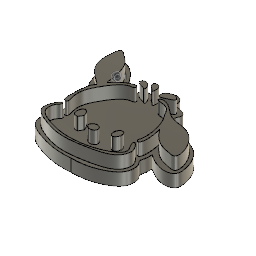
pochacco v3 (Autodesk Fusion 360 design; units mm, degrees)
Autodesk Fusion 360 part; units mm, degrees
(part 1 of 2)
sketch "Sketch1" plane through (0, 0, 0) normal (0, 0, 1) x (1, 0, 0)
  spline S0 degree 5 poles (-0.6709, -13.445) (-0.783, -13.4498) (-1.0072, -13.459) (-1.3442, -13.4715) (-1.7958, -13.4859) (-2.365, -13.4975) (-2.9391, -13.4984) (-3.5187, -13.4833) (-4.106, -13.4469) (-4.7062, -13.3844) (-5.3283, -13.2926) (-5.9822, -13.1694) (-6.6768, -13.0129) (-7.4173, -12.8216) (-8.2027, -12.5932) (-9.0235, -12.3247) (-9.8597, -12.0116) (-10.6769, -11.6473) (-11.4304, -11.2245) (-12.0725, -10.7371) (-12.5591, -10.1826) (-12.8561, -9.5641) (-12.9463, -8.892) (-12.8356, -8.1865) (-12.5616, -7.4801) (-12.1923, -6.8157) (-11.8085, -6.235) (-11.4898, -5.7696) (-11.2987, -5.4297) (-11.2671, -5.1966) (-11.3773, -5.0079) (-11.5611, -4.7626) (-11.7362, -4.3632) (-11.8325, -3.7477) (-11.8251, -2.9297) (-11.7255, -1.9782) (-11.5691, -0.9945) (-11.4045, -0.0892) (-11.2826, 0.6397) (-11.2442, 1.1314) (-11.3109, 1.3806) (-11.4696, 1.4712) (-11.6758, 1.5583) (-11.8871, 1.7597) (-12.0894, 2.0706) (-12.2879, 2.4194) (-12.4965, 2.7197) (-12.728, 2.9335) (-12.9875, 3.0981) (-13.2749, 3.2834) (-13.5856, 3.566) (-13.912, 3.9925) (-14.2441, 4.5797) (-14.5698, 5.3213) (-14.8753, 6.1921) (-15.1462, 7.1536) (-15.3673, 8.1587) (-15.5233, 9.1573) (-15.5998, 10.1003) (-15.5828, 10.9464) (-15.4608, 11.6626) (-15.2255, 12.2237) (-14.8731, 12.6119) (-14.4066, 12.8168) (-13.8357, 12.8345) (-13.1799, 12.6674) (-12.4665, 12.3245) (-11.7278, 11.8208) (-10.9984, 11.1782) (-10.3118, 10.4256) (-9.698, 9.5988) (-9.1805, 8.7406) (-8.7731, 7.9018) (-8.4778, 7.1402) (-8.2807, 6.5221) (-8.1557, 6.1073) (-8.0671, 5.9319) (-7.9735, 5.9948) (-7.8294, 6.2361) (-7.593, 6.5406) (-7.2472, 6.7929) (-6.8148, 6.9181) (-6.383, 6.9377) (-6.0614, 6.9338) (-5.9338, 7.0029) (-6.0018, 7.2066) (-6.1645, 7.543) (-6.2897, 7.972) (-6.2688, 8.4304) (-6.0758, 8.8508) (-5.7419, 9.1752) (-5.3303, 9.3696) (-4.9133, 9.4359) (-4.5448, 9.4322) (-4.2529, 9.4431) (-4.0374, 9.5402) (-3.8635, 9.7382) (-3.6665, 9.976) (-3.3863, 10.167) (-2.9979, 10.2378) (-2.5366, 10.1656) (-2.0673, 9.9643) (-1.6593, 9.6771) (-1.3617, 9.3669) (-1.1717, 9.1088) (-1.0427, 8.9709) (-0.9073, 8.9925) (-0.6976, 9.157) (-0.3587, 9.4027) (0.1403, 9.6505) (0.7963, 9.8245) (1.5579, 9.8797) (2.3378, 9.8023) (3.0366, 9.6007) (3.5622, 9.2992) (3.8526, 8.9306) (3.8934, 8.5294) (3.7467, 8.1242) (3.5327, 7.7352) (3.3803, 7.3754) (3.3923, 7.0507) (3.5931, 6.7603) (3.9282, 6.4983) (4.3136, 6.2565) (4.6678, 6.0275) (4.9601, 5.8076) (5.2168, 5.597) (5.4892, 5.3975) (5.8342, 5.2103) (6.2852, 5.0334) (6.85, 4.8615) (7.5179, 4.6873) (8.2646, 4.5017) (9.0581, 4.2949) (9.8636, 4.057) (10.6488, 3.7787) (11.3903, 3.4522) (12.0729, 3.0716) (12.6879, 2.6335) (13.2319, 2.1373) (13.7056, 1.5858) (14.1121, 0.9858) (14.4558, 0.3482) (14.7408, -0.3111) (14.9701, -0.9713) (15.1451, -1.61) (15.2662, -2.2059) (15.332, -2.7413) (15.3397, -3.2051) (15.2847, -3.5952) (15.1607, -3.9217) (14.9606, -4.1992) (14.6768, -4.4397) (14.3026, -4.644) (13.8328, -4.7975) (13.2671, -4.8789) (12.6118, -4.8662) (11.8835, -4.7446) (11.1103, -4.5126) (10.3365, -4.1907) (9.6195, -3.8228) (9.017, -3.4646) (8.5761, -3.1758) (8.321, -3.0107) (8.2437, -3.0092) (8.2866, -3.1872) (8.3535, -3.5308) (8.3608, -4.0006) (8.2888, -4.5302) (8.1739, -5.0419) (8.076, -5.4679) (8.0543, -5.7687) (8.1385, -5.9551) (8.3064, -6.1019) (8.5111, -6.3) (8.7096, -6.603) (8.8732, -7.0146) (8.9811, -7.5114) (9.0199, -8.0542) (8.9803, -8.6054) (8.8551, -9.142) (8.6396, -9.6517) (8.3323, -10.1301) (7.9349, -10.5777) (7.4531, -10.9973) (6.897, -11.39) (6.2807, -11.7543) (5.6208, -12.0873) (4.9348, -12.3852) (4.24, -12.6443) (3.5517, -12.8619) (2.8818, -13.0371) (2.2375, -13.1714) (1.6203, -13.2697) (1.0271, -13.3388) (0.4523, -13.3865) (0.0014, -13.4134) (-0.3348, -13.4302) (-0.5588, -13.4402) (-0.6709, -13.445) knots 0 0 0 0 0 0 0.00512821 0.01025641 0.01538462 0.02051282 0.02564103 0.03076923 0.03589744 0.04102564 0.04615385 0.05128205 0.05641026 0.06153846 0.06666667 0.07179487 0.07692308 0.08205128 0.08717949 0.09230769 0.0974359 0.1025641 0.10769231 0.11282051 0.11794872 0.12307692 0.12820513 0.13333333 0.13846154 0.14358974 0.14871795 0.15384615 0.15897436 0.16410256 0.16923077 0.17435897 0.17948718 0.18461538 0.18974359 0.19487179 0.2 0.20512821 0.21025641 0.21538462 0.22051282 0.22564103 0.23076923 0.23589744 0.24102564 0.24615385 0.25128205 0.25641026 0.26153846 0.26666667 0.27179487 0.27692308 0.28205128 0.28717949 0.29230769 0.2974359 0.3025641 0.30769231 0.31282051 0.31794872 0.32307692 0.32820513 0.33333333 0.33846154 0.34358974 0.34871795 0.35384615 0.35897436 0.36410256 0.36923077 0.37435897 0.37948718 0.38461538 0.38974359 0.39487179 0.4 0.40512821 0.41025641 0.41538462 0.42051282 0.42564103 0.43076923 0.43589744 0.44102564 0.44615385 0.45128205 0.45641026 0.46153846 0.46666667 0.47179487 0.47692308 0.48205128 0.48717949 0.49230769 0.4974359 0.5025641 0.50769231 0.51282051 0.51794872 0.52307692 0.52820513 0.53333333 0.53846154 0.54358974 0.54871795 0.55384615 0.55897436 0.56410256 0.56923077 0.57435897 0.57948718 0.58461538 0.58974359 0.59487179 0.6 0.60512821 0.61025641 0.61538462 0.62051282 0.62564103 0.63076923 0.63589744 0.64102564 0.64615385 0.65128205 0.65641026 0.66153846 0.66666667 0.67179487 0.67692308 0.68205128 0.68717949 0.69230769 0.6974359 0.7025641 0.70769231 0.71282051 0.71794872 0.72307692 0.72820513 0.73333333 0.73846154 0.74358974 0.74871795 0.75384615 0.75897436 0.76410256 0.76923077 0.77435897 0.77948718 0.78461538 0.78974359 0.79487179 0.8 0.80512821 0.81025641 0.81538462 0.82051282 0.82564103 0.83076923 0.83589744 0.84102564 0.84615385 0.85128205 0.85641026 0.86153846 0.86666667 0.87179487 0.87692308 0.88205128 0.88717949 0.89230769 0.8974359 0.9025641 0.90769231 0.91282051 0.91794872 0.92307692 0.92820513 0.93333333 0.93846154 0.94358974 0.94871795 0.95384615 0.95897436 0.96410256 0.96923077 0.97435897 0.97948718 0.98461538 0.98974359 0.99487179 1 1 1 1 1 1
  point P0 (-4.0523, -13.445)
  point P1 (-9.3122, -12.2106)
  point P2 (-12.8546, -8.4535)
  point P3 (-11.2981, -5.2868)
  point P4 (-11.7275, -4.267)
  point P5 (-11.2981, 1.2613)
  point P6 (-11.6738, 1.5833)
  point P7 (-12.4253, 2.6031)
  point P8 (-13.3377, 3.3545)
  point P9 (-15.5383, 9.4732)
  point P10 (-14.1428, 12.801)
  point P11 (-8.7755, 7.8631)
  point P12 (-8, 6)
  point P13 (-7.1653, 6.7896)
  point P14 (-6, 7)
  point P15 (-6.2529, 7.9704)
  point P16 (-5.2331, 9.3659)
  point P17 (-4.106, 9.5269)
  point P18 (-3.4082, 10.1173)
  point P19 (-1.5833, 9.5806)
  point P20 (-1, 9)
  point P21 (0.3489, 9.6879)
  point P22 (3.8376, 8.7755)
  point P23 (3.4082, 7.219)
  point P24 (4.4817, 6.1455)
  point P25 (5.6088, 5.3404)
  point P26 (10, 4)
  point P27 (14.3575, 0.5099)
  point P28 (15.3236, -3.1935)
  point P29 (14.7332, -4.3743)
  point P30 (11.4055, -4.589)
  point P31 (8.2924, -3.0325)
  point P32 (8.3461, -3.6766)
  point P33 (8.0778, -5.7162)
  point P34 (8.3998, -6.1992)
  point P35 (9, -8)
  point P36 (7.6484, -10.8151)
  point P37 (3, -13)
sketch "Sketch2" plane through (0, 0, 0) normal (0, 0, 1) x (1, 0, 0)
  line L0 (-5, -6) -> (-5.5551, -6.9506)
  spline S0 degree 5 poles (-5, -6) (-4.9873, -6.0708) (-4.971, -6.2073) (-4.9739, -6.3935) (-5.0334, -6.5992) (-5.1932, -6.7885) (-5.4235, -6.9202) (-5.703, -7.002) (-6.0043, -7.0264) (-6.297, -6.972) (-6.5506, -6.8162) (-6.7385, -6.5461) (-6.8412, -6.1684) (-6.8505, -5.7228) (-6.7682, -5.2711) (-6.6041, -4.8826) (-6.3745, -4.621) (-6.1008, -4.5319) (-5.8082, -4.6262) (-5.5241, -4.8758) (-5.2754, -5.2304) (-5.1244, -5.5494) (-5.0469, -5.7823) (-5.0127, -5.9292) (-5, -6) knots 0 0 0 0 0 0 0.05 0.1 0.15 0.2 0.25 0.3 0.35 0.4 0.45 0.5 0.55 0.6 0.65 0.7 0.75 0.8 0.85 0.9 0.95 1 1 1 1 1 1
  point P0 (-6.7359, -6.4753)
  point P1 (-6.1992, -4.589)
sketch "Sketch3" plane through (0, 0, 0) normal (0, 0, 1) x (1, 0, 0)
  spline S0 degree 5 poles (2.1201, -6.3602) (2.1016, -6.3367) (2.0689, -6.2938) (2.0317, -6.2416) (2.003, -6.1859) (1.9929, -6.0963) (2.0011, -5.9456) (2.0273, -5.7181) (2.079, -5.4308) (2.1668, -5.1203) (2.3002, -4.8333) (2.4835, -4.6168) (2.7117, -4.5083) (2.9662, -4.5253) (3.2203, -4.6685) (3.4438, -4.9245) (3.6088, -5.2681) (3.6945, -5.665) (3.6932, -6.0738) (3.6098, -6.4503) (3.4578, -6.754) (3.2564, -6.9526) (3.0276, -7.0286) (2.7933, -6.9844) (2.572, -6.8496) (2.3783, -6.6692) (2.2537, -6.5259) (2.1795, -6.4352) (2.1385, -6.3838) (2.1201, -6.3602) knots 0 0 0 0 0 0 0.04 0.08 0.12 0.16 0.2 0.24 0.28 0.32 0.36 0.4 0.44 0.48 0.52 0.56 0.6 0.64 0.68 0.72 0.76 0.8 0.84 0.88 0.92 0.96 1 1 1 1 1 1
  spline S1 degree 5 poles (-1.3687, -8.0778) (-1.4057, -8.0896) (-1.4798, -8.1125) (-1.5911, -8.1441) (-1.7386, -8.1767) (-1.9212, -8.1873) (-2.1006, -8.1533) (-2.2732, -8.0641) (-2.4307, -7.917) (-2.5593, -7.7201) (-2.6431, -7.4883) (-2.6676, -7.2406) (-2.6223, -6.9973) (-2.5042, -6.777) (-2.3206, -6.5934) (-2.0868, -6.456) (-1.8224, -6.3704) (-1.5487, -6.3386) (-1.2858, -6.3594) (-1.0491, -6.4285) (-0.8479, -6.5391) (-0.687, -6.6827) (-0.5678, -6.8493) (-0.49, -7.0283) (-0.4527, -7.2092) (-0.4557, -7.3821) (-0.4983, -7.5387) (-0.5789, -7.6734) (-0.6943, -7.7842) (-0.8387, -7.8742) (-1.0044, -7.9495) (-1.1476, -8.0032) (-1.2577, -8.0415) (-1.3316, -8.0659) (-1.3687, -8.0778) knots 0 0 0 0 0 0 0.033333 0.066667 0.1 0.133333 0.166667 0.2 0.233333 0.266667 0.3 0.333333 0.366667 0.4 0.433333 0.466667 0.5 0.533333 0.566667 0.6 0.633333 0.666667 0.7 0.733333 0.766667 0.8 0.833333 0.866667 0.9 0.933333 0.966667 1 1 1 1 1 1
  spline S2 degree 5 poles (-10, 2) (-10.0186, 2.0485) (-10.069, 2.1405) (-10.1839, 2.2654) (-10.4088, 2.4137) (-10.7729, 2.59) (-11.1764, 2.7771) (-11.5819, 2.9925) (-11.9682, 3.2495) (-12.3265, 3.5579) (-12.6567, 3.9245) (-12.9634, 4.3535) (-13.2526, 4.8472) (-13.5278, 5.4061) (-13.79, 6.0285) (-14.0377, 6.7091) (-14.2669, 7.4384) (-14.4708, 8.2018) (-14.6403, 8.9783) (-14.7636, 9.7401) (-14.826, 10.451) (-14.8115, 11.0694) (-14.7061, 11.5548) (-14.5002, 11.8734) (-14.1909, 12.0038) (-13.7859, 11.9431) (-13.3038, 11.7103) (-12.771, 11.3384) (-12.2177, 10.8682) (-11.6748, 10.3418) (-11.17, 9.7955) (-10.7246, 9.254) (-10.3499, 8.7227) (-10.0484, 8.1935) (-9.816, 7.6518) (-9.644, 7.0825) (-9.5211, 6.4772) (-9.4351, 5.8403) (-9.3756, 5.1968) (-9.3339, 4.5929) (-9.3001, 4.0833) (-9.2609, 3.7215) (-9.1974, 3.5491) (-9.0816, 3.585) (-8.8769, 3.8179) (-8.5525, 4.2132) (-8.0941, 4.7177) (-7.5191, 5.2648) (-6.8724, 5.7825) (-6.2138, 6.2037) (-5.6084, 6.475) (-5.1161, 6.5669) (-4.7812, 6.4823) (-4.6214, 6.2685) (-4.62, 6.0193) (-4.7442, 5.8262) (-4.9631, 5.7204) (-5.2561, 5.6645) (-5.608, 5.5945) (-6.0083, 5.4519) (-6.4492, 5.2073) (-6.9239, 4.8502) (-7.4251, 4.386) (-7.944, 3.8304) (-8.4681, 3.2048) (-8.9805, 2.5312) (-9.4575, 1.8275) (-9.8727, 1.1074) (-10.2004, 0.382) (-10.42, -0.3397) (-10.5193, -1.05) (-10.4991, -1.7411) (-10.376, -2.4049) (-10.1877, -3.0316) (-9.9939, -3.6092) (-9.8584, -4.1238) (-9.8338, -4.5594) (-9.9446, -4.8985) (-10.1731, -5.1223) (-10.4379, -5.2096) (-10.6397, -5.15) (-10.7214, -4.9593) (-10.7167, -4.6912) (-10.6977, -4.4052) (-10.7214, -4.1315) (-10.7948, -3.8513) (-10.8982, -3.5264) (-10.9976, -3.1177) (-11.063, -2.6127) (-11.0729, -2.0241) (-11.0143, -1.3806) (-10.8849, -0.7203) (-10.6939, -0.083) (-10.4631, 0.4963) (-10.2298, 0.9968) (-10.0408, 1.4121) (-9.9613, 1.6796) (-9.9574, 1.8495) (-9.9814, 1.9515) (-10, 2) knots 0 0 0 0 0 0 0.01052632 0.02105263 0.03157895 0.04210526 0.05263158 0.06315789 0.07368421 0.08421053 0.09473684 0.10526316 0.11578947 0.12631579 0.13684211 0.14736842 0.15789474 0.16842105 0.17894737 0.18947368 0.2 0.21052632 0.22105263 0.23157895 0.24210526 0.25263158 0.26315789 0.27368421 0.28421053 0.29473684 0.30526316 0.31578947 0.32631579 0.33684211 0.34736842 0.35789474 0.36842105 0.37894737 0.38947368 0.4 0.41052632 0.42105263 0.43157895 0.44210526 0.45263158 0.46315789 0.47368421 0.48421053 0.49473684 0.50526316 0.51578947 0.52631579 0.53684211 0.54736842 0.55789474 0.56842105 0.57894737 0.58947368 0.6 0.61052632 0.62105263 0.63157895 0.64210526 0.65263158 0.66315789 0.67368421 0.68421053 0.69473684 0.70526316 0.71578947 0.72631579 0.73684211 0.74736842 0.75789474 0.76842105 0.77894737 0.78947368 0.8 0.81052632 0.82105263 0.83157895 0.84210526 0.85263158 0.86315789 0.87368421 0.88421053 0.89473684 0.90526316 0.91578947 0.92631579 0.93684211 0.94736842 0.95789474 0.96842105 0.97894737 0.98947368 1 1 1 1 1 1
  spline S3 degree 5 poles (1, 6) (0.9263, 6.0109) (0.7895, 6.0343) (0.6205, 6.0771) (0.4842, 6.1578) (0.4887, 6.306) (0.668, 6.4812) (0.9946, 6.6344) (1.4281, 6.7112) (1.9261, 6.6683) (2.4575, 6.4946) (3.0012, 6.2043) (3.5444, 5.829) (4.0813, 5.41) (4.6112, 4.9909) (5.1372, 4.6101) (5.6643, 4.2919) (6.1984, 4.0456) (6.7457, 3.8685) (7.3116, 3.7479) (7.9003, 3.6638) (8.5133, 3.5904) (9.1491, 3.4994) (9.8027, 3.3614) (10.4661, 3.1491) (11.1286, 2.8397) (11.7772, 2.4174) (12.3971, 1.8764) (12.9722, 1.2226) (13.485, 0.4774) (13.9176, -0.321) (14.2533, -1.1246) (14.4786, -1.8814) (14.5849, -2.5424) (14.5707, -3.0681) (14.4432, -3.4348) (14.2199, -3.6411) (13.9316, -3.7154) (13.6114, -3.7012) (13.2853, -3.6437) (12.9596, -3.573) (12.6234, -3.5017) (12.2587, -3.4296) (11.8475, -3.346) (11.3819, -3.2332) (10.8645, -3.0705) (10.3054, -2.8387) (9.7219, -2.525) (9.136, -2.1272) (8.5732, -1.6582) (8.061, -1.1516) (7.626, -0.6569) (7.2904, -0.231) (7.0689, 0.0691) (6.9653, 0.194) (6.9691, 0.1095) (7.0534, -0.1966) (7.1826, -0.7135) (7.318, -1.4065) (7.4251, -2.2144) (7.4779, -3.0523) (7.4606, -3.8283) (7.368, -4.4571) (7.2077, -4.8751) (7.0005, -5.0541) (6.783, -5.0174) (6.6072, -4.851) (6.5178, -4.6493) (6.5225, -4.4413) (6.5897, -4.1849) (6.6736, -3.8184) (6.7343, -3.3035) (6.747, -2.642) (6.6972, -1.8607) (6.5805, -1.0045) (6.4002, -0.1272) (6.1658, 0.717) (5.891, 1.4828) (5.5925, 2.1418) (5.2881, 2.6922) (4.9938, 3.1506) (4.7223, 3.5442) (4.4794, 3.9025) (4.2626, 4.2496) (4.0577, 4.5955) (3.8386, 4.9308) (3.5766, 5.2374) (3.2488, 5.4951) (2.8457, 5.6895) (2.3805, 5.8212) (1.8841, 5.9021) (1.4961, 5.9422) (1.2317, 5.9692) (1.0737, 5.9891) (1, 6) knots 0 0 0 0 0 0 0.01111111 0.02222222 0.03333333 0.04444444 0.05555556 0.06666667 0.07777778 0.08888889 0.1 0.11111111 0.12222222 0.13333333 0.14444444 0.15555556 0.16666667 0.17777778 0.18888889 0.2 0.21111111 0.22222222 0.23333333 0.24444444 0.25555556 0.26666667 0.27777778 0.28888889 0.3 0.31111111 0.32222222 0.33333333 0.34444444 0.35555556 0.36666667 0.37777778 0.38888889 0.4 0.41111111 0.42222222 0.43333333 0.44444444 0.45555556 0.46666667 0.47777778 0.48888889 0.5 0.51111111 0.52222222 0.53333333 0.54444444 0.55555556 0.56666667 0.57777778 0.58888889 0.6 0.61111111 0.62222222 0.63333333 0.64444444 0.65555556 0.66666667 0.67777778 0.68888889 0.7 0.71111111 0.72222222 0.73333333 0.74444444 0.75555556 0.76666667 0.77777778 0.78888889 0.8 0.81111111 0.82222222 0.83333333 0.84444444 0.85555556 0.86666667 0.87777778 0.88888889 0.9 0.91111111 0.92222222 0.93333333 0.94444444 0.95555556 0.96666667 0.97777778 0.98888889 1 1 1 1 1 1
  point P0 (2, -6)
  point P1 (2.4958, -4.6427)
  point P2 (3.6229, -5.3941)
  point P3 (3, -7)
  point P4 (-2.2274, -8.0778)
  point P5 (-2.6031, -7)
  point P6 (-1.3687, -6.3602)
  point P7 (-0.5099, -7)
  point P8 (-0.6172, -7.702)
  point P9 (-11.1371, 2.7641)
  point P10 (-12.962, 4.3743)
  point P11 (-14.6795, 9.2586)
  point P12 (-14.2501, 11.9422)
  point P13 (-11.1371, 9.7416)
  point P14 (-9.4732, 6.0919)
  point P15 (-9.2049, 3.6229)
  point P16 (-8.3998, 4.3743)
  point P17 (-4.8574, 6.4676)
  point P18 (-4.6964, 5.9308)
  point P19 (-5.5015, 5.6088)
  point P20 (-8.5071, 3.1399)
  point P21 (-10.3857, -2.2811)
  point P22 (-10, -4.9111)
  point P23 (-10.6004, -5.1258)
  point P24 (-10.7077, -4.4817)
  point P25 (-10.9224, -3.4082)
  point P26 (-10.6004, 0.1342)
  point P27 (0.5099, 6.2529)
  point P28 (1.476, 6.6823)
  point P29 (4.8037, 4.8574)
  point P30 (8.2388, 3.6229)
  point P31 (12.9083, 1.2613)
  point P32 (14.4111, -3.4082)
  point P33 (13.4987, -3.6766)
  point P34 (12.1569, -3.4082)
  point P35 (9, -2)
  point P36 (7.0043, 0.1342)
  point P37 (7.2727, -1.2076)
  point P38 (7, -5)
  point P39 (6.5749, -4.75)
  point P40 (6.6286, -3.9986)
  point P41 (5.8772, 1.476)
  point P42 (4.3207, 4.1596)
  point P43 (3.1935, 5.5015)
sketch "Sketch4" plane through (0, 0, 0) normal (0, 0, 1) x (1, 0, 0)
sketch "Sketch5" plane through (0, 0, 0) normal (0, 0, 1) x (1, 0, 0)
  spline S0 degree 5 poles (-3.5692, 6.8433) (-3.6043, 6.856) (-3.6794, 6.8823) (-3.8061, 6.9223) (-4.0002, 6.9732) (-4.272, 7.0356) (-4.5557, 7.1066) (-4.8314, 7.1988) (-5.078, 7.3226) (-5.2745, 7.4814) (-5.4018, 7.6695) (-5.4448, 7.8747) (-5.3954, 8.08) (-5.2543, 8.2649) (-5.0345, 8.4072) (-4.7587, 8.4857) (-4.4547, 8.4836) (-4.1514, 8.3912) (-3.8746, 8.2093) (-3.6428, 7.9535) (-3.4638, 7.6549) (-3.3387, 7.3522) (-3.2642, 7.085) (-3.2356, 6.8859) (-3.2489, 6.7742) (-3.3043, 6.7465) (-3.3855, 6.7726) (-3.4687, 6.8057) (-3.5341, 6.8305) (-3.5692, 6.8433) knots 0 0 0 0 0 0 0.04 0.08 0.12 0.16 0.2 0.24 0.28 0.32 0.36 0.4 0.44 0.48 0.52 0.56 0.6 0.64 0.68 0.72 0.76 0.8 0.84 0.88 0.92 0.96 1 1 1 1 1 1
  spline S1 degree 5 poles (-2.3348, 7.5947) (-2.3755, 7.6122) (-2.4586, 7.6494) (-2.5874, 7.7111) (-2.7608, 7.8038) (-2.9617, 7.9396) (-3.128, 8.1) (-3.2436, 8.2888) (-3.2975, 8.5047) (-3.2869, 8.7372) (-3.2163, 8.9686) (-3.0952, 9.1773) (-2.9362, 9.3413) (-2.7532, 9.4415) (-2.5592, 9.4651) (-2.3659, 9.4068) (-2.1834, 9.2683) (-2.0206, 9.0585) (-1.8846, 8.7938) (-1.7808, 8.498) (-1.7131, 8.1995) (-1.6841, 7.927) (-1.6952, 7.7058) (-1.7467, 7.5539) (-1.8384, 7.4776) (-1.9688, 7.4687) (-2.1017, 7.5032) (-2.2144, 7.5446) (-2.2941, 7.5772) (-2.3348, 7.5947) knots 0 0 0 0 0 0 0.04 0.08 0.12 0.16 0.2 0.24 0.28 0.32 0.36 0.4 0.44 0.48 0.52 0.56 0.6 0.64 0.68 0.72 0.76 0.8 0.84 0.88 0.92 0.96 1 1 1 1 1 1
  spline S2 degree 5 poles (-0.2415, 7.2727) (-0.2716, 7.2959) (-0.3244, 7.3456) (-0.3814, 7.43) (-0.4115, 7.5603) (-0.373, 7.7488) (-0.2632, 7.9577) (-0.0918, 8.1792) (0.1256, 8.402) (0.3705, 8.613) (0.6245, 8.7989) (0.8722, 8.9479) (1.1039, 9.0515) (1.3196, 9.1067) (1.5282, 9.1159) (1.7407, 9.0844) (1.9647, 9.0188) (2.199, 8.9248) (2.4265, 8.805) (2.6201, 8.6599) (2.7501, 8.4903) (2.7903, 8.2982) (2.7263, 8.0891) (2.5597, 7.8731) (2.3032, 7.6623) (1.9778, 7.4699) (1.6089, 7.3081) (1.2229, 7.1869) (0.8434, 7.1119) (0.4905, 7.0845) (0.1808, 7.1032) (-0.022, 7.1524) (-0.1442, 7.2064) (-0.2115, 7.2495) (-0.2415, 7.2727) knots 0 0 0 0 0 0 0.033333 0.066667 0.1 0.133333 0.166667 0.2 0.233333 0.266667 0.3 0.333333 0.366667 0.4 0.433333 0.466667 0.5 0.533333 0.566667 0.6 0.633333 0.666667 0.7 0.733333 0.766667 0.8 0.833333 0.866667 0.9 0.933333 0.966667 1 1 1 1 1 1
  spline S3 degree 5 poles (-12.0495, 5.7162) (-12.0629, 5.7109) (-12.0919, 5.7054) (-12.1416, 5.7122) (-12.217, 5.7515) (-12.3166, 5.8483) (-12.4109, 5.9864) (-12.4901, 6.1555) (-12.5463, 6.3409) (-12.5746, 6.5236) (-12.5732, 6.6829) (-12.5427, 6.7996) (-12.486, 6.8588) (-12.4086, 6.8526) (-12.3176, 6.7838) (-12.2219, 6.6625) (-12.1304, 6.5043) (-12.0521, 6.3272) (-11.9944, 6.1493) (-11.9628, 5.9865) (-11.9604, 5.8515) (-11.9825, 5.7742) (-12.0117, 5.7367) (-12.0362, 5.7214) (-12.0495, 5.7162) knots 0 0 0 0 0 0 0.05 0.1 0.15 0.2 0.25 0.3 0.35 0.4 0.45 0.5 0.55 0.6 0.65 0.7 0.75 0.8 0.85 0.9 0.95 1 1 1 1 1 1
  spline S4 degree 5 poles (-11.1908, 6.5749) (-11.2139, 6.5864) (-11.261, 6.6157) (-11.3333, 6.6778) (-11.428, 6.7927) (-11.5301, 6.9681) (-11.6027, 7.1489) (-11.6354, 7.3088) (-11.622, 7.4261) (-11.5636, 7.4898) (-11.469, 7.5013) (-11.3514, 7.4697) (-11.2258, 7.4074) (-11.1067, 7.326) (-11.005, 7.2321) (-10.9276, 7.1277) (-10.8787, 7.0133) (-10.8601, 6.8911) (-10.8721, 6.7667) (-10.9138, 6.6532) (-10.9833, 6.5694) (-11.0581, 6.5406) (-11.1223, 6.5466) (-11.1677, 6.5634) (-11.1908, 6.5749) knots 0 0 0 0 0 0 0.05 0.1 0.15 0.2 0.25 0.3 0.35 0.4 0.45 0.5 0.55 0.6 0.65 0.7 0.75 0.8 0.85 0.9 0.95 1 1 1 1 1 1
  spline S5 degree 5 poles (-11.9422, 8.3998) (-11.9584, 8.3921) (-11.9936, 8.3798) (-12.0541, 8.3713) (-12.1463, 8.3815) (-12.27, 8.436) (-12.3903, 8.5354) (-12.4959, 8.678) (-12.5771, 8.8539) (-12.6261, 9.0426) (-12.6383, 9.2187) (-12.6115, 9.3563) (-12.5474, 9.4342) (-12.451, 9.4402) (-12.332, 9.3774) (-12.2028, 9.2594) (-12.0771, 9.1063) (-11.9682, 8.9403) (-11.8873, 8.7815) (-11.842, 8.6427) (-11.8356, 8.5303) (-11.8613, 8.4632) (-11.8964, 8.4261) (-11.926, 8.4075) (-11.9422, 8.3998) knots 0 0 0 0 0 0 0.05 0.1 0.15 0.2 0.25 0.3 0.35 0.4 0.45 0.5 0.55 0.6 0.65 0.7 0.75 0.8 0.85 0.9 0.95 1 1 1 1 1 1
  spline S6 degree 5 poles (-13.284, 9.7416) (-13.303, 9.7417) (-13.3412, 9.7442) (-13.3988, 9.7546) (-13.4718, 9.7822) (-13.5469, 9.8393) (-13.5967, 9.9177) (-13.6147, 10.0137) (-13.5983, 10.1199) (-13.5501, 10.2245) (-13.4765, 10.3138) (-13.3862, 10.3745) (-13.2894, 10.3965) (-13.1956, 10.3753) (-13.1132, 10.3149) (-13.049, 10.2254) (-13.0078, 10.12) (-12.993, 10.0128) (-13.0057, 9.916) (-13.045, 9.8372) (-13.1079, 9.7804) (-13.1731, 9.7534) (-13.2275, 9.7436) (-13.2651, 9.7415) (-13.284, 9.7416) knots 0 0 0 0 0 0 0.05 0.1 0.15 0.2 0.25 0.3 0.35 0.4 0.45 0.5 0.55 0.6 0.65 0.7 0.75 0.8 0.85 0.9 0.95 1 1 1 1 1 1
  spline S7 degree 5 poles (7.6484, 1.3687) (7.6156, 1.3787) (7.5486, 1.4013) (7.4449, 1.4432) (7.3068, 1.5155) (7.1543, 1.6314) (7.0421, 1.7688) (6.9865, 1.9208) (6.9971, 2.0777) (7.072, 2.2262) (7.1986, 2.3508) (7.3579, 2.4361) (7.5284, 2.4699) (7.6904, 2.4453) (7.8299, 2.3638) (7.9418, 2.2368) (8.0262, 2.0812) (8.0872, 1.9163) (8.1298, 1.7602) (8.1582, 1.6267) (8.1732, 1.5207) (8.1728, 1.4413) (8.1534, 1.384) (8.1106, 1.3442) (8.0402, 1.3199) (7.9397, 1.3126) (7.8352, 1.3229) (7.7451, 1.3413) (7.6811, 1.3587) (7.6484, 1.3687) knots 0 0 0 0 0 0 0.04 0.08 0.12 0.16 0.2 0.24 0.28 0.32 0.36 0.4 0.44 0.48 0.52 0.56 0.6 0.64 0.68 0.72 0.76 0.8 0.84 0.88 0.92 0.96 1 1 1 1 1 1
  spline S8 degree 5 poles (10.1173, 0.6709) (10.1051, 0.6727) (10.0792, 0.6727) (10.0354, 0.6631) (9.9673, 0.6381) (9.8721, 0.6152) (9.7774, 0.6296) (9.6963, 0.7018) (9.6421, 0.8318) (9.6265, 0.9991) (9.6582, 1.1721) (9.7409, 1.316) (9.8726, 1.4) (10.0428, 1.4063) (10.2321, 1.3356) (10.4169, 1.2009) (10.5732, 1.0242) (10.6803, 0.832) (10.7247, 0.6509) (10.705, 0.5034) (10.6345, 0.4042) (10.535, 0.3601) (10.4303, 0.3699) (10.3398, 0.4244) (10.2713, 0.5057) (10.2197, 0.5895) (10.1831, 0.6403) (10.1526, 0.6621) (10.1296, 0.6691) (10.1173, 0.6709) knots 0 0 0 0 0 0 0.04 0.08 0.12 0.16 0.2 0.24 0.28 0.32 0.36 0.4 0.44 0.48 0.52 0.56 0.6 0.64 0.68 0.72 0.76 0.8 0.84 0.88 0.92 0.96 1 1 1 1 1 1
  spline S9 degree 5 poles (10.3857, -1.2076) (10.3583, -1.196) (10.3083, -1.1721) (10.2489, -1.1346) (10.199, -1.0806) (10.1662, -1.0001) (10.1396, -0.9003) (10.1017, -0.7802) (10.0548, -0.6507) (10.0216, -0.5346) (10.0313, -0.4572) (10.1085, -0.4401) (10.2615, -0.4935) (10.4712, -0.609) (10.7022, -0.7668) (10.9114, -0.9402) (11.0574, -1.1012) (11.1095, -1.226) (11.0571, -1.3003) (10.9193, -1.3245) (10.7318, -1.308) (10.5759, -1.2736) (10.4728, -1.2419) (10.4131, -1.2193) (10.3857, -1.2076) knots 0 0 0 0 0 0 0.05 0.1 0.15 0.2 0.25 0.3 0.35 0.4 0.45 0.5 0.55 0.6 0.65 0.7 0.75 0.8 0.85 0.9 0.95 1 1 1 1 1 1
  spline S10 degree 5 poles (11.4055, -0.4562) (11.3841, -0.4553) (11.343, -0.4544) (11.2864, -0.4562) (11.2221, -0.4632) (11.1585, -0.4721) (11.1084, -0.4715) (11.0689, -0.4531) (11.0404, -0.4128) (11.027, -0.3527) (11.0342, -0.2788) (11.0674, -0.1998) (11.1298, -0.1255) (11.2202, -0.0656) (11.3335, -0.0284) (11.4617, -0.0199) (11.5951, -0.0432) (11.7227, -0.0969) (11.8336, -0.1745) (11.9175, -0.2642) (11.9658, -0.3522) (11.9731, -0.4254) (11.9379, -0.4742) (11.8638, -0.4956) (11.7605, -0.4946) (11.6404, -0.4804) (11.5415, -0.467) (11.471, -0.4599) (11.4268, -0.4571) (11.4055, -0.4562) knots 0 0 0 0 0 0 0.04 0.08 0.12 0.16 0.2 0.24 0.28 0.32 0.36 0.4 0.44 0.48 0.52 0.56 0.6 0.64 0.68 0.72 0.76 0.8 0.84 0.88 0.92 0.96 1 1 1 1 1 1
  spline S11 degree 5 poles (12.6936, -1.798) (12.6701, -1.7856) (12.6229, -1.7591) (12.5532, -1.7148) (12.467, -1.6488) (12.381, -1.5596) (12.3257, -1.4685) (12.3073, -1.3807) (12.3282, -1.3027) (12.3862, -1.2432) (12.4744, -1.2112) (12.5837, -1.2144) (12.703, -1.2566) (12.8209, -1.3361) (12.9263, -1.4432) (13.0096, -1.5639) (13.0629, -1.682) (13.0806, -1.782) (13.0607, -1.8521) (13.0051, -1.8867) (12.9195, -1.8867) (12.8337, -1.8625) (12.7643, -1.8336) (12.7172, -1.8104) (12.6936, -1.798) knots 0 0 0 0 0 0 0.05 0.1 0.15 0.2 0.25 0.3 0.35 0.4 0.45 0.5 0.55 0.6 0.65 0.7 0.75 0.8 0.85 0.9 0.95 1 1 1 1 1 1
  spline S12 degree 5 poles (-10.3857, -5.7698) (-10.3398, -5.7371) (-10.2551, -5.6872) (-10.1508, -5.6596) (-10.0569, -5.7193) (-10.0064, -5.9255) (-10.0252, -6.1836) (-10.1183, -6.4064) (-10.2816, -6.5568) (-10.4939, -6.6865) (-10.7234, -6.8783) (-10.9336, -7.1979) (-11.0889, -7.6457) (-11.1589, -8.1793) (-11.1218, -8.7333) (-10.969, -9.2401) (-10.7084, -9.6494) (-10.3693, -9.9511) (-9.993, -10.1641) (-9.6211, -10.3237) (-9.2858, -10.4689) (-8.9976, -10.6294) (-8.7386, -10.816) (-8.4751, -11.0267) (-8.1668, -11.251) (-7.7782, -11.4751) (-7.2864, -11.6854) (-6.6784, -11.8686) (-5.9504, -12.0123) (-5.1065, -12.1059) (-4.1574, -12.1411) (-3.1196, -12.1121) (-2.0138, -12.0165) (-0.8638, -11.856) (0.3042, -11.6367) (1.4634, -11.3679) (2.5862, -11.0615) (3.6461, -10.7299) (4.6178, -10.386) (5.4787, -10.041) (6.2093, -9.7039) (6.7943, -9.3803) (7.2236, -9.0707) (7.4929, -8.7704) (7.605, -8.4666) (7.571, -8.1435) (7.4135, -7.7872) (7.1682, -7.3922) (6.8868, -6.9665) (6.6278, -6.5302) (6.4454, -6.1132) (6.3805, -5.7536) (6.4498, -5.4952) (6.6361, -5.3856) (6.9011, -5.4575) (7.2025, -5.7034) (7.5022, -6.073) (7.7678, -6.4984) (7.9755, -6.9141) (8.112, -7.2761) (8.1777, -7.5874) (8.1833, -7.8838) (8.143, -8.2069) (8.0695, -8.581) (7.9678, -8.9874) (7.8376, -9.382) (7.6752, -9.7166) (7.4763, -9.9563) (7.2384, -10.1048) (6.9614, -10.1985) (6.6459, -10.2847) (6.2927, -10.4028) (5.9016, -10.5677) (5.4721, -10.7775) (5.0039, -11.0186) (4.4967, -11.272) (3.9514, -11.5184) (3.3699, -11.7451) (2.7549, -11.9447) (2.1105, -12.1144) (1.441, -12.2547) (0.7517, -12.3681) (0.0478, -12.4583) (-0.665, -12.529) (-1.3809, -12.5823) (-2.0946, -12.6192) (-2.8005, -12.6394) (-3.4937, -12.6418) (-4.1696, -12.625) (-4.8239, -12.5871) (-5.4531, -12.5265) (-6.0545, -12.4419) (-6.6261, -12.3327) (-7.1669, -12.1987) (-7.6771, -12.0405) (-8.1586, -11.859) (-8.6144, -11.6558) (-9.0498, -11.4329) (-9.4716, -11.1927) (-9.8858, -10.9372) (-10.2952, -10.6669) (-10.6966, -10.38) (-11.0787, -10.0718) (-11.4182, -9.733) (-11.6848, -9.3524) (-11.8484, -8.9214) (-11.8868, -8.4379) (-11.7922, -7.9099) (-11.5798, -7.361) (-11.2855, -6.8274) (-10.9549, -6.351) (-10.6992, -6.0492) (-10.5305, -5.8833) (-10.4316, -5.8025) (-10.3857, -5.7698) knots 0 0 0 0 0 0 0.00909091 0.01818182 0.02727273 0.03636364 0.04545455 0.05454545 0.06363636 0.07272727 0.08181818 0.09090909 0.1 0.10909091 0.11818182 0.12727273 0.13636364 0.14545455 0.15454545 0.16363636 0.17272727 0.18181818 0.19090909 0.2 0.20909091 0.21818182 0.22727273 0.23636364 0.24545455 0.25454545 0.26363636 0.27272727 0.28181818 0.29090909 0.3 0.30909091 0.31818182 0.32727273 0.33636364 0.34545455 0.35454545 0.36363636 0.37272727 0.38181818 0.39090909 0.4 0.40909091 0.41818182 0.42727273 0.43636364 0.44545455 0.45454545 0.46363636 0.47272727 0.48181818 0.49090909 0.5 0.50909091 0.51818182 0.52727273 0.53636364 0.54545455 0.55454545 0.56363636 0.57272727 0.58181818 0.59090909 0.6 0.60909091 0.61818182 0.62727273 0.63636364 0.64545455 0.65454545 0.66363636 0.67272727 0.68181818 0.69090909 0.7 0.70909091 0.71818182 0.72727273 0.73636364 0.74545455 0.75454545 0.76363636 0.77272727 0.78181818 0.79090909 0.8 0.80909091 0.81818182 0.82727273 0.83636364 0.84545455 0.85454545 0.86363636 0.87272727 0.88181818 0.89090909 0.9 0.90909091 0.91818182 0.92727273 0.93636364 0.94545455 0.95454545 0.96363636 0.97272727 0.98181818 0.99090909 1 1 1 1 1 1
  point P0 (-4.9647, 7.2727)
  point P1 (-5.3404, 8.1314)
  point P2 (-3.945, 8.2388)
  point P3 (-3.2472, 6.8433)
  point P4 (-3.2472, 8.3461)
  point P5 (-2.8715, 9.3659)
  point P6 (-2, 9)
  point P7 (-1.7444, 7.5947)
  point P8 (-0.2415, 7.9704)
  point P9 (1, 9)
  point P10 (2, 9)
  point P11 (2.7641, 8.3461)
  point P12 (1.476, 7.2727)
  point P13 (-12.4789, 6.1455)
  point P14 (-12.4789, 6.8433)
  point P15 (-12.0495, 6.3066)
  point P16 (-11.6202, 7.38)
  point P17 (-11.1908, 7.38)
  point P18 (-10.8687, 6.8433)
  point P19 (-12.4789, 8.6682)
  point P20 (-12.5326, 9.4196)
  point P21 (-11.9422, 8.8828)
  point P22 (-13.6061, 10.01)
  point P23 (-13.284, 10.3857)
  point P24 (-13, 10)
  point P25 (7, 2)
  point P26 (7.6484, 2.4421)
  point P27 (8.1314, 1.7444)
  point P28 (8.1314, 1.3687)
  point P29 (9.7416, 0.6709)
  point P30 (9.849, 1.3687)
  point P31 (10.7077, 0.6709)
  point P32 (10.3857, 0.4025)
  point P33 (10.1173, -0.8319)
  point P34 (10.1173, -0.4562)
  point P35 (11.0834, -1.2076)
  point P36 (11.0834, -0.4562)
  point P37 (11.0834, -0.1879)
  point P38 (11.6738, -0.0805)
  point P39 (11.9422, -0.4562)
  point P40 (12.3179, -1.3687)
  point P41 (12.6936, -1.2613)
  point P42 (13.0693, -1.798)
  point P43 (-10.0636, -5.7698)
  point P44 (-10.1173, -6.3602)
  point P45 (-10.7077, -6.897)
  point P46 (-10.9224, -9.2586)
  point P47 (-9.3659, -10.4394)
  point P48 (-8.2388, -11.1908)
  point P49 (-2, -12)
  point P50 (7.2727, -8.9902)
  point P51 (7.38, -7.7557)
  point P52 (6.4139, -5.7698)
  point P53 (6.7896, -5.4478)
  point P54 (8, -7)
  point P55 (8.1314, -8.2388)
  point P56 (7.5947, -9.7953)
  point P57 (6.6823, -10.2783)
  point P58 (4.428, -11.2981)
  point P59 (-0.1879, -12.4789)
  point P60 (-5.3404, -12.5326)
  point P61 (-8.5608, -11.6738)
  point P62 (-10.8151, -10.2783)
  point P63 (-11.8349, -8.2388)
extrude "Extrude1" add sketch "Sketch5" along normal blind 3 contours S0 makes body 1
extrude "Extrude2" add sketch "Sketch3" along normal blind 3 separate body contours S3 makes body 2
extrude "Extrude3" add sketch "Sketch2" along normal blind 3 separate body contours L0 S0 picked at (-5.8647, -6.3423) makes body 3
sketch "Sketch6" plane through (0, 0, 0) normal (0, 0, 1) x (1, 0, 0)
  spline S0 degree 5 poles (-10, 2) (-10.01, 2.036) (-10.0453, 2.1108) (-10.1474, 2.2349) (-10.3859, 2.4339) (-10.8347, 2.7499) (-11.393, 3.1342) (-12.0076, 3.5812) (-12.6229, 4.0819) (-13.1891, 4.627) (-13.6733, 5.2111) (-14.0597, 5.8323) (-14.3455, 6.4896) (-14.5375, 7.1809) (-14.6486, 7.9014) (-14.6949, 8.6414) (-14.692, 9.3839) (-14.6517, 10.1032) (-14.5784, 10.7623) (-14.471, 11.3191) (-14.3252, 11.735) (-14.1362, 11.9825) (-13.9007, 12.0521) (-13.6202, 11.9628) (-13.3012, 11.7594) (-12.9526, 11.4943) (-12.5846, 11.2134) (-12.206, 10.9382) (-11.8235, 10.6576) (-11.4425, 10.342) (-11.068, 9.9532) (-10.7055, 9.4558) (-10.3621, 8.8276) (-10.047, 8.0724) (-9.7717, 7.2242) (-9.5468, 6.3366) (-9.3788, 5.4754) (-9.2683, 4.7097) (-9.2065, 4.1044) (-9.1724, 3.7107) (-9.1314, 3.5595) (-9.029, 3.6505) (-8.804, 3.9529) (-8.4136, 4.4136) (-7.8609, 4.9623) (-7.1905, 5.5211) (-6.4714, 6.0135) (-5.7845, 6.3744) (-5.2082, 6.559) (-4.8035, 6.5535) (-4.6023, 6.3818) (-4.5875, 6.1225) (-4.7071, 5.8806) (-4.9057, 5.7334) (-5.1562, 5.676) (-5.452, 5.6487) (-5.794, 5.5768) (-6.1761, 5.4127) (-6.5828, 5.1473) (-6.9941, 4.7946) (-7.3893, 4.384) (-7.7508, 3.9497) (-8.0681, 3.5212) (-8.3413, 3.1136) (-8.5775, 2.7318) (-8.7882, 2.3723) (-8.9859, 2.0258) (-9.1813, 1.6798) (-9.3801, 1.3213) (-9.5834, 0.938) (-9.7877, 0.5199) (-9.9851, 0.061) (-10.1642, -0.4399) (-10.3094, -0.9769) (-10.405, -1.5388) (-10.4387, -2.1108) (-10.405, -2.676) (-10.3098, -3.2174) (-10.1726, -3.7193) (-10.0326, -4.169) (-9.9371, -4.5561) (-9.9267, -4.87) (-10.0234, -5.0985) (-10.2124, -5.225) (-10.4434, -5.2306) (-10.6607, -5.1043) (-10.8309, -4.853) (-10.9445, -4.4982) (-11.0055, -4.0669) (-11.0259, -3.5855) (-11.0179, -3.0709) (-10.9923, -2.533) (-10.9576, -1.978) (-10.9188, -1.4115) (-10.8765, -0.8411) (-10.8256, -0.2797) (-10.7543, 0.2508) (-10.6494, 0.7257) (-10.5042, 1.1234) (-10.3248, 1.4329) (-10.1363, 1.6588) (-10.0217, 1.7964) (-9.9855, 1.8949) (-9.99, 1.964) (-10, 2) knots 0 0 0 0 0 0 0.01 0.02 0.03 0.04 0.05 0.06 0.07 0.08 0.09 0.1 0.11 0.12 0.13 0.14 0.15 0.16 0.17 0.18 0.19 0.2 0.21 0.22 0.23 0.24 0.25 0.26 0.27 0.28 0.29 0.3 0.31 0.32 0.33 0.34 0.35 0.36 0.37 0.38 0.39 0.4 0.41 0.42 0.43 0.44 0.45 0.46 0.47 0.48 0.49 0.5 0.51 0.52 0.53 0.54 0.55 0.56 0.57 0.58 0.59 0.6 0.61 0.62 0.63 0.64 0.65 0.66 0.67 0.68 0.69 0.7 0.71 0.72 0.73 0.74 0.75 0.76 0.77 0.78 0.79 0.8 0.81 0.82 0.83 0.84 0.85 0.86 0.87 0.88 0.89 0.9 0.91 0.92 0.93 0.94 0.95 0.96 0.97 0.98 0.99 1 1 1 1 1 1
  point P0 (-12.801, 4.267)
  point P1 (-14.6795, 9.4732)
  point P2 (-14, 12)
  point P3 (-12.6936, 11.2981)
  point P4 (-10.493, 9.0439)
  point P5 (-9.1512, 3.6766)
  point P6 (-8.6682, 4.106)
  point P7 (-4.75, 6.4676)
  point P8 (-4.75, 5.8772)
  point P9 (-5.6088, 5.6088)
  point P10 (-7.702, 3.9986)
  point P11 (-9, 2)
  point P12 (-10, 0)
  point P13 (-10.2783, -3.3009)
  point P14 (-10, -5)
  point P15 (-10.493, -5.1794)
  point P16 (-11, -4)
  point P17 (-10.8687, -0.7783)
  point P18 (-10.2783, 1.476)
extrude "Extrude4" add sketch "Sketch6" along normal blind 3 separate body makes body 4
sketch "Sketch7" plane through (0, 0, 0) normal (0, 0, 1) x (1, 0, 0)
  spline S0 degree 5 poles (-2.6031, 7.9704) (-2.6346, 7.9941) (-2.7003, 8.0402) (-2.8068, 8.1048) (-2.9593, 8.1837) (-3.146, 8.2807) (-3.3038, 8.3886) (-3.4098, 8.5182) (-3.447, 8.6736) (-3.4105, 8.8477) (-3.3062, 9.0239) (-3.147, 9.1814) (-2.9499, 9.299) (-2.7334, 9.3594) (-2.5136, 9.3537) (-2.304, 9.282) (-2.1152, 9.1506) (-1.9554, 8.9707) (-1.8304, 8.7561) (-1.7433, 8.5216) (-1.6951, 8.2816) (-1.6844, 8.0493) (-1.7079, 7.8373) (-1.7602, 7.6565) (-1.8342, 7.5166) (-1.9209, 7.4253) (-2.0107, 7.3879) (-2.0962, 7.4055) (-2.1751, 7.4739) (-2.2532, 7.5816) (-2.3418, 7.7119) (-2.4309, 7.8204) (-2.5117, 7.8978) (-2.5717, 7.9467) (-2.6031, 7.9704) knots 0 0 0 0 0 0 0.033333 0.066667 0.1 0.133333 0.166667 0.2 0.233333 0.266667 0.3 0.333333 0.366667 0.4 0.433333 0.466667 0.5 0.533333 0.566667 0.6 0.633333 0.666667 0.7 0.733333 0.766667 0.8 0.833333 0.866667 0.9 0.933333 0.966667 1 1 1 1 1 1
  spline S1 degree 5 poles (-0.1879, 7.9704) (-0.1651, 8.0236) (-0.1127, 8.1288) (-0.0145, 8.2815) (0.1505, 8.4695) (0.3928, 8.6711) (0.649, 8.8363) (0.8999, 8.9645) (1.1327, 9.056) (1.3474, 9.109) (1.5548, 9.1205) (1.7679, 9.0879) (1.9955, 9.0109) (2.2349, 8.893) (2.4648, 8.7438) (2.654, 8.5757) (2.7693, 8.4013) (2.784, 8.2307) (2.6874, 8.0683) (2.4886, 7.9117) (2.209, 7.7561) (1.8773, 7.5965) (1.524, 7.4315) (1.1753, 7.2662) (0.848, 7.1154) (0.5519, 6.9989) (0.2926, 6.9377) (0.0733, 6.9485) (-0.102, 7.0404) (-0.2264, 7.2089) (-0.2901, 7.4367) (-0.2857, 7.6474) (-0.2492, 7.8099) (-0.2106, 7.9173) (-0.1879, 7.9704) knots 0 0 0 0 0 0 0.033333 0.066667 0.1 0.133333 0.166667 0.2 0.233333 0.266667 0.3 0.333333 0.366667 0.4 0.433333 0.466667 0.5 0.533333 0.566667 0.6 0.633333 0.666667 0.7 0.733333 0.766667 0.8 0.833333 0.866667 0.9 0.933333 0.966667 1 1 1 1 1 1
  point P0 (-3.4082, 8.5608)
  point P1 (-2.8715, 9.3122)
  point P2 (-1.8517, 8.7755)
  point P3 (-1.798, 7.5947)
  point P4 (-2.1201, 7.4337)
  point P5 (1, 9)
  point P6 (2, 9)
  point P7 (2.7641, 8.2924)
  point P8 (1.5297, 7.4337)
  point P9 (0, 7)
extrude "Extrude5" add sketch "Sketch7" along normal blind 3 separate body contours S1 makes body 5
sketch "Sketch8" plane through (0, 0, 0) normal (0, 0, 1) x (1, 0, 0)
  spline S0 degree 5 poles (-2.6568, 7.8631) (-2.6953, 7.8921) (-2.772, 7.9484) (-2.8852, 8.0273) (-3.0274, 8.1223) (-3.1793, 8.2345) (-3.2947, 8.3544) (-3.3652, 8.4941) (-3.3848, 8.6583) (-3.3514, 8.8381) (-3.2663, 9.0161) (-3.1342, 9.1712) (-2.9634, 9.2832) (-2.7654, 9.3383) (-2.5547, 9.3331) (-2.347, 9.2713) (-2.1572, 9.1614) (-1.997, 9.0139) (-1.8734, 8.8386) (-1.7867, 8.6421) (-1.7319, 8.4293) (-1.7018, 8.2049) (-1.6893, 7.9757) (-1.689, 7.7516) (-1.7005, 7.5485) (-1.728, 7.3863) (-1.778, 7.284) (-1.8566, 7.2545) (-1.9673, 7.2994) (-2.1089, 7.4057) (-2.2766, 7.5516) (-2.4255, 7.6805) (-2.541, 7.7744) (-2.6183, 7.8341) (-2.6568, 7.8631) knots 0 0 0 0 0 0 0.033333 0.066667 0.1 0.133333 0.166667 0.2 0.233333 0.266667 0.3 0.333333 0.366667 0.4 0.433333 0.466667 0.5 0.533333 0.566667 0.6 0.633333 0.666667 0.7 0.733333 0.766667 0.8 0.833333 0.866667 0.9 0.933333 0.966667 1 1 1 1 1 1
  point P0 (-3.3545, 8.5071)
  point P1 (-2.9788, 9.2586)
  point P2 (-2, 9)
  point P3 (-1.6907, 7.8631)
  point P4 (-1.8517, 7.2727)
extrude "Extrude6" add sketch "Sketch8" along normal blind 3 separate body makes body 6
sketch "Sketch9" plane through (0, 0, 0) normal (0, 0, 1) x (1, 0, 0)
  spline S0 degree 5 poles (2.7641, -6.897) (2.7136, -6.906) (2.6132, -6.9126) (2.4675, -6.8873) (2.2919, -6.7846) (2.1215, -6.5566) (2.0143, -6.253) (1.979, -5.9039) (2.0187, -5.5426) (2.13, -5.2031) (2.3042, -4.9174) (2.5274, -4.7132) (2.7812, -4.611) (3.0426, -4.6214) (3.2849, -4.7423) (3.4812, -4.9614) (3.6078, -5.258) (3.6483, -5.6047) (3.5975, -5.9692) (3.4636, -6.316) (3.2638, -6.6104) (3.0698, -6.7793) (2.9167, -6.8582) (2.8147, -6.8879) (2.7641, -6.897) knots 0 0 0 0 0 0 0.05 0.1 0.15 0.2 0.25 0.3 0.35 0.4 0.45 0.5 0.55 0.6 0.65 0.7 0.75 0.8 0.85 0.9 0.95 1 1 1 1 1 1
  point P0 (2, -6)
  point P1 (2.7641, -4.6427)
  point P2 (3.6229, -5.5015)
extrude "Extrude7" add sketch "Sketch9" along normal blind 3 separate body makes body 7
sketch "Sketch10" plane through (0, 0, 0) normal (0, 0, 1) x (1, 0, 0)
  spline S0 degree 5 poles (-2, -8) (-2.0408, -7.9847) (-2.1215, -7.9515) (-2.2388, -7.8934) (-2.3822, -7.7987) (-2.5224, -7.6479) (-2.6058, -7.4628) (-2.6178, -7.2467) (-2.5509, -7.0115) (-2.407, -6.7785) (-2.195, -6.5726) (-1.9298, -6.4191) (-1.6308, -6.3382) (-1.3211, -6.3412) (-1.0257, -6.4261) (-0.7697, -6.5807) (-0.5747, -6.7864) (-0.4571, -7.0213) (-0.4247, -7.2632) (-0.474, -7.4933) (-0.591, -7.6973) (-0.7571, -7.8649) (-0.9523, -7.9897) (-1.1599, -8.0696) (-1.3709, -8.1063) (-1.5823, -8.1045) (-1.751, -8.0767) (-1.8766, -8.0431) (-1.9592, -8.0153) (-2, -8) knots 0 0 0 0 0 0 0.04 0.08 0.12 0.16 0.2 0.24 0.28 0.32 0.36 0.4 0.44 0.48 0.52 0.56 0.6 0.64 0.68 0.72 0.76 0.8 0.84 0.88 0.92 0.96 1 1 1 1 1 1
  point P0 (-2.6031, -7.3263)
  point P1 (-1.637, -6.3602)
  point P2 (-0.4562, -7.1116)
  point P3 (-1, -8)
extrude "Extrude8" add sketch "Sketch10" along normal blind 3 separate body makes body 8
sketch "Sketch11" plane through (0, 0, 0) normal (0, 0, 1) x (1, 0, 0)
  spline S0 degree 5 poles (-10.4394, -5.8235) (-10.3931, -5.7881) (-10.3072, -5.7354) (-10.2004, -5.7112) (-10.1035, -5.785) (-10.0524, -6.0062) (-10.0679, -6.2608) (-10.1457, -6.4583) (-10.276, -6.5881) (-10.4422, -6.7232) (-10.6238, -6.9388) (-10.798, -7.2554) (-10.9418, -7.6564) (-11.033, -8.1055) (-11.0519, -8.5657) (-10.9829, -9.0135) (-10.8159, -9.4338) (-10.5477, -9.8191) (-10.183, -10.1666) (-9.737, -10.4763) (-9.232, -10.7498) (-8.6932, -10.9903) (-8.1445, -11.2016) (-7.6044, -11.3882) (-7.0817, -11.5544) (-6.5725, -11.7038) (-6.064, -11.8395) (-5.5378, -11.9626) (-4.9738, -12.0728) (-4.3532, -12.1672) (-3.6623, -12.2402) (-2.8937, -12.2836) (-2.046, -12.2882) (-1.1234, -12.2444) (-0.1362, -12.1433) (0.8999, -11.9781) (1.9636, -11.7445) (3.028, -11.4421) (4.0609, -11.0754) (5.0246, -10.655) (5.8791, -10.1958) (6.5871, -9.7149) (7.1181, -9.2293) (7.4527, -8.7537) (7.5871, -8.2979) (7.5371, -7.8656) (7.3442, -7.4499) (7.0721, -7.0381) (6.7926, -6.6227) (6.575, -6.2119) (6.4734, -5.8389) (6.5142, -5.5763) (6.6952, -5.5032) (6.9871, -5.6548) (7.3363, -5.9913) (7.6804, -6.4335) (7.9627, -6.8924) (8.1447, -7.2973) (8.2249, -7.6326) (8.2277, -7.927) (8.1839, -8.225) (8.1112, -8.5625) (7.9999, -8.9459) (7.8259, -9.3632) (7.5619, -9.7916) (7.1885, -10.2065) (6.7064, -10.5903) (6.1327, -10.9327) (5.495, -11.2287) (4.8255, -11.4786) (4.1554, -11.6858) (3.5096, -11.8567) (2.9001, -11.9989) (2.324, -12.1204) (1.769, -12.2289) (1.2172, -12.3309) (0.6494, -12.4306) (0.0486, -12.5293) (-0.5947, -12.6243) (-1.2817, -12.7088) (-2.0075, -12.7742) (-2.7633, -12.8105) (-3.5375, -12.8087) (-4.3183, -12.7612) (-5.0947, -12.6639) (-5.8593, -12.5171) (-6.6085, -12.3265) (-7.3404, -12.1002) (-8.0535, -11.8474) (-8.7448, -11.5763) (-9.4085, -11.292) (-10.0336, -10.9948) (-10.603, -10.6783) (-11.0915, -10.3274) (-11.4718, -9.9244) (-11.7195, -9.4547) (-11.8193, -8.9124) (-11.7697, -8.3061) (-11.5905, -7.6658) (-11.3195, -7.0395) (-11.0033, -6.4823) (-10.7528, -6.1345) (-10.585, -5.9477) (-10.4857, -5.8589) (-10.4394, -5.8235) knots 0 0 0 0 0 0 0.01 0.02 0.03 0.04 0.05 0.06 0.07 0.08 0.09 0.1 0.11 0.12 0.13 0.14 0.15 0.16 0.17 0.18 0.19 0.2 0.21 0.22 0.23 0.24 0.25 0.26 0.27 0.28 0.29 0.3 0.31 0.32 0.33 0.34 0.35 0.36 0.37 0.38 0.39 0.4 0.41 0.42 0.43 0.44 0.45 0.46 0.47 0.48 0.49 0.5 0.51 0.52 0.53 0.54 0.55 0.56 0.57 0.58 0.59 0.6 0.61 0.62 0.63 0.64 0.65 0.66 0.67 0.68 0.69 0.7 0.71 0.72 0.73 0.74 0.75 0.76 0.77 0.78 0.79 0.8 0.81 0.82 0.83 0.84 0.85 0.86 0.87 0.88 0.89 0.9 0.91 0.92 0.93 0.94 0.95 0.96 0.97 0.98 0.99 1 1 1 1 1 1
  point P0 (-10.1173, -5.8235)
  point P1 (-10.1173, -6.3602)
  point P2 (-10.4394, -6.7359)
  point P3 (-11, -8)
  point P4 (-10.4394, -9.9026)
  point P5 (-7.702, -11.3518)
  point P6 (-4.75, -12.1032)
  point P7 (3.2472, -11.3518)
  point P8 (7.541, -8.0778)
  point P9 (6.5749, -6.1455)
  point P10 (6.6823, -5.5551)
  point P11 (8, -7)
  point P12 (8.1851, -8.1851)
  point P13 (7.4874, -9.849)
  point P14 (3.7839, -11.7812)
  point P15 (0.3489, -12.4789)
  point P16 (-4.8037, -12.6936)
  point P17 (-10, -11)
  point P18 (-11.7812, -8.6682)
extrude "Extrude9" add sketch "Sketch11" along normal blind 3 separate body makes body 9
sketch "Sketch12" plane through (0, 0, 0) normal (0, 0, 1) x (1, 0, 0)
  spline S0 degree 5 poles (-11.9959, 8.3998) (-12.0216, 8.4027) (-12.0741, 8.4142) (-12.1548, 8.4483) (-12.2619, 8.5253) (-12.3852, 8.6608) (-12.4898, 8.8183) (-12.5687, 8.9791) (-12.6162, 9.1255) (-12.6267, 9.2443) (-12.5963, 9.3276) (-12.5235, 9.371) (-12.4112, 9.3734) (-12.268, 9.3359) (-12.1096, 9.2614) (-11.9548, 9.1547) (-11.8232, 9.0226) (-11.7318, 8.8745) (-11.692, 8.7224) (-11.7062, 8.5817) (-11.7688, 8.4691) (-11.8489, 8.4138) (-11.9198, 8.3968) (-11.9702, 8.3969) (-11.9959, 8.3998) knots 0 0 0 0 0 0 0.05 0.1 0.15 0.2 0.25 0.3 0.35 0.4 0.45 0.5 0.55 0.6 0.65 0.7 0.75 0.8 0.85 0.9 0.95 1 1 1 1 1 1
  spline S1 degree 5 poles (-11.9959, 8.3998) (-12.0216, 8.4027) (-12.0741, 8.4142) (-12.1548, 8.4483) (-12.2619, 8.5253) (-12.3852, 8.6608) (-12.4898, 8.8183) (-12.5687, 8.9791) (-12.6162, 9.1255) (-12.6267, 9.2443) (-12.5963, 9.3276) (-12.5235, 9.371) (-12.4112, 9.3734) (-12.268, 9.3359) (-12.1096, 9.2614) (-11.9548, 9.1547) (-11.8232, 9.0226) (-11.7318, 8.8745) (-11.692, 8.7224) (-11.7062, 8.5817) (-11.7688, 8.4691) (-11.8489, 8.4138) (-11.9198, 8.3968) (-11.9702, 8.3969) (-11.9959, 8.3998) knots 0 0 0 0 0 0 0.05 0.1 0.15 0.2 0.25 0.3 0.35 0.4 0.45 0.5 0.55 0.6 0.65 0.7 0.75 0.8 0.85 0.9 0.95 1 1 1 1 1 1
  point P0 (-12.5863, 9.0439)
  point P1 (-12.4253, 9.3659)
  point P2 (-11.7275, 8.8292)
  point P3 (-12.5863, 9.0439)
  point P4 (-12.4253, 9.3659)
  point P5 (-11.7275, 8.8292)
  constraint coincident P3 P0
  constraint coincident P4 P1
  constraint coincident P5 P2
extrude "Extrude10" add sketch "Sketch1" along normal blind 0 and the other way blind 3 bodies 1 2 3 4 5 6 7 8 9
sketch "Sketch13" plane through (0, 0, 0) normal (0, 0, 1) x (1, 0, 0)
  circle A0 centre (-0.8856, 10.654) radius 1.6111
extrude "Extrude11" add sketch "Sketch13" along normal blind 0 and the other way blind 3 bodies 1